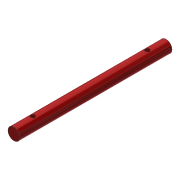
# Autodesk Inventor part: COXA_ROLL_SHAFT_D4
Saved by Autodesk Inventor 2019.4 (Build 234330000, 330)
## iProperties
Created: 2019-11-06
Part Number: COXA_ROLL_SHAFT_D4
Material: 一般
Document SubType Name: Modeling
Designer: y6tada
Density: 1 g/cm^3
Appearance: 滑らか - 赤
Author: y6tada
Autodesk Inventor part; units mm, degrees
ref_plane "YZ Plane" through (0, 0, 0) normal (1, 0, 0) x (0, 1, 0)
ref_plane "XZ Plane" through (0, 0, 0) normal (0, 1, 0) x (-1, 0, 0)
ref_plane "XY Plane" through (0, 0, 0) normal (0, 0, 1) x (1, 0, 0)
sketch "スケッチ1" plane through (0, 0, 0) normal (0, 0, 1) x (1, 0, 0)
  circle A0 centre (0, 0) radius 2
  dimension "d0" = 4
  constraints: 1 centre point, 1 coincident
  measures "d0" diameter of A0
extrude "押し出し1" add sketch "スケッチ1" along normal mid plane 48
chamfer "面取り1" distance 0.1 angle 45 2 edges at (-2, 0, 24) (-2, 0, -24)
sketch "スケッチ2" plane through (0, 0, 0) normal (0, 1, 0) x (-1, 0, 0)
  line L0 (0, 0) -> (3.4806, 0) construction
  line L1 (0, 0) -> (0, -21.75) construction
  circle A0 centre (0, -21.75) radius 0.75
  circle A1 centre (0, 21.75) radius 0.75
  line L2 (2.6688, -21) -> (-4.3603, -21) construction
  dimension "d6" = 1.5
  dimension "d11" = 42
  constraints: 6 end point, 2 centre point, 2 horizontal, 1 coincident, 1 symmetric about line, 1 tangent, 1 vertical, 1 other
  measures "d6" diameter of A0
  measures "d11" diameter of L2 L0
extrude "押し出し2" cut sketch "スケッチ2" along normal through all both and the other way through all
